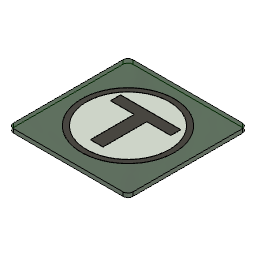
mbta_coaster (Autodesk Fusion 360 design; units mm, degrees)
part number: 2026-06-30-18-54-41-195
Autodesk Fusion 360 part; units mm, degrees
sketch "Sketch1" plane through (0, 0, 0) normal (0, 0, 1) x (1, 0, 0)
  line L0 (0, 0) -> (95.25, 0)
  line L1 (95.25, 0) -> (95.25, 95.25)
  line L2 (95.25, 95.25) -> (0, 95.25)
  line L3 (0, 95.25) -> (0, 0)
  dimension "d1" = 95.25
  dimension "d2" = 95.25
  constraint horizontal L0
  constraint vertical L1
  constraint horizontal L2
  constraint vertical L3
  constraint coincident L0.start L3.end
  measures "d1" distance of L0.start L0.end
  measures "d2" distance of L0.start L2.end
extrude "Extrude1" add sketch "Sketch1" along normal blind 3.2
sketch "Sketch2" plane through (0, 0, 3.2) normal (0, 0, 1) x (-1, 0, 0)
  line L0 (0, -95.25) -> (0, 0)
  line L1 (0, 0) -> (-95.25, 0)
  line L2 (-95.25, 0) -> (-95.25, -95.25)
  line L3 (-95.25, -95.25) -> (0, -95.25)
  circle A0 centre (-47.625, -47.625) radius 33
  circle A1 centre (-47.625, -47.625) radius 37
  line L4 (-23.4439, -57.8934) -> (-23.4439, -65.8934)
  line L5 (-23.4439, -65.8934) -> (-71.4439, -65.8934)
  line L6 (-71.4439, -65.8934) -> (-71.4439, -57.8934)
  line L7 (-42.3445, -22.9899) -> (-52.3445, -22.9899)
  line L8 (-52.3445, -22.9899) -> (-52.3445, -57.8934)
  line L9 (-42.3445, -57.8934) -> (-42.3445, -22.9899)
  line L10 (-71.4439, -57.8934) -> (-52.3445, -57.8934)
  line L11 (-42.3445, -57.8934) -> (-23.4439, -57.8934)
  point P0 (-47.625, -68.4053)
  point P1 (-47.625, -47.625)
  dimension "d5" = 66
  dimension "d6" = 4
  dimension "d9" = 48
  dimension "d10" = 8
  constraint horizontal L10
  constraint perpendicular L4 L11
  constraint parallel L5 L10
  constraint parallel L4 L6
  constraint horizontal L7
  constraint perpendicular L7 L8
  constraint parallel L8 L9
  constraint coincident P1 A0.centre
  constraint collinear L10 L11
  measures "d5" diameter of A0
  measures "d9" distance of L4.end L5.end
  measures "d10" distance of L4.start L4.end
fillet "Fillet1" radius 4 1 edges at (0, 0, 1.6)
fillet "Fillet2" radius 4 1 edges at (95.25, 0, 1.6)
fillet "Fillet3" radius 4 1 edges at (95.25, 95.25, 1.6)
fillet "Fillet4" radius 4 1 edges at (0, 95.25, 1.6)
extrude "Extrude2" add sketch "Sketch2" along normal blind 0.1 contours A1 | L4 L5 L6 L7 L8 L9 L10 L11
extrude "Extrude3" cut 1 faces at (59.86, 36.6396, 3.2) along direction (0, 0, -1) blind 0.01
extrude "Extrude4" cut 1 faces at (59.86, 36.6396, 3.19) along direction (0, 0, -1) blind 0.01
